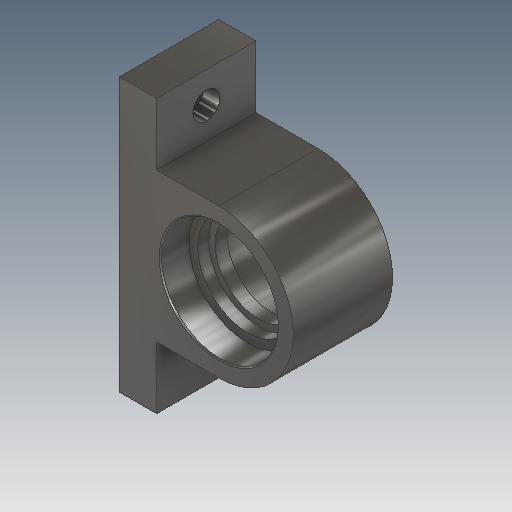
# Autodesk Inventor part: shoulder_joint_fit_v2
Saved by Autodesk Inventor 2021.4 (Build 254397000, 397)
## iProperties
Created: 2020-05-06
Part Number: shoulder_joint_fit_v2
Material: Stahl, hochfest, niedrig legiert
Document SubType Name: Modeling
Designer: Alex
Density: 7.85 g/cm^3
Appearance: Stahl - poliert
Mass: 965.569 g
Surface Area: 266.743 cm^2
Volume: 123.002 cm^3
Author: Alex
Autodesk Inventor part; units mm, degrees
ref_plane "YZ Plane" through (0, 0, 0) normal (1, 0, 0) x (0, 1, 0)
ref_plane "XZ Plane" through (0, 0, 0) normal (0, 1, 0) x (-1, 0, 0)
sketch "Skizze1" plane through (0, 0, 0) normal (0, 0, 1) x (1, 0, 0)
  line L0 (0, 0) -> (55, 0)
  line L1 (55, 0) -> (55, 60)
  line L2 (55, 60) -> (0, 60)
  line L3 (0, 60) -> (0, 0)
  dimension "d0" = 60
  dimension "d1" = 55
  constraints: 8 end point, 2 parallel, 1 horizontal, 1 perpendicular
  measures "d0" distance between parallel lines of L0 L2
  measures "d1" distance of L1.end L2.end
extrude "Grundkörper" add sketch "Skizze1" along normal blind 40
fillet "Konturverrundung" radius 30 2 edges at (55, 60, 20) (55, 0, 20)
sketch "Skizze2" plane through (0, 0, 40) normal (0, 0, 1) x (1, 0, 0)
  point P0 (0, 0)
  point P1 (25, 30)
  point P2 (25, 30)
  constraints: 1 coincident
hole "Durchgangsbohrung 60H7" at (25, 30, 40) direction (0, 0, -1) diameter 55 end through all
sketch "Skizze3" plane through (0, 0, 0) normal (-1, 0, 0) x (0, 0, 1)
  line L0 (0, 0) -> (40, 0) construction
  line L1 (40, 60) -> (40, 0) construction
  line L2 (0, 0) -> (40, 60) construction
  line L3 (0, 60) -> (40, 60) construction
  line L4 (0, 60) -> (40, 0) construction
  line L5 (0, 85) -> (40, 85)
  line L6 (40, 85) -> (40, -25)
  line L7 (40, -25) -> (0, -25)
  line L8 (0, -25) -> (0, 85)
  line L9 (0, 85) -> (40, -25) construction
  line L10 (40, 85) -> (0, -25) construction
  point P0 (20, 30)
  dimension "d16" = 110
  constraints: 16 end point, 3 midpoint, 2 parallel, 1 collinear, 1 horizontal, 1 perpendicular
  measures "d16" distance of L5.end L6.end
extrude "Aufnahmeplatte" add sketch "Skizze3" along normal blind 15
sketch "Skizze4" plane through (0, 0, 0) normal (1, 0, 0) x (0, 0, -1)
  line L0 (-40, 85) -> (0, 85) projected
  line L1 (-20, 85) -> (-20, -25)
  line L2 (-40, -25) -> (0, -25) projected
  line L3 (0, 60) -> (-40, 60) projected
  line L4 (8, 30) -> (-48, 30) projected
  point P0 (0, 0)
  point P1 (-20, 72.5)
  point P2 (-20, -12.5)
  dimension "d26" = 25
  dimension "d27" = 12.5
  constraints: 2 end point, 2 midpoint, 1 point on line, 1 symmetric about line
  measures "d26" distance between parallel lines of L0 L3
  measures "d27" distance from line of point (-20, 72.5) L0
hole "Senkung_Zylinderkopfschraube M6" at (0, 72.5, 20) at (0, -12.5, 20) direction (-1, 0, 0) diameter 6.6 end through all counterbore diameter 11 counterbore depth 6.6 clearance for "Inbusschraube DIN EN ISO 4762" size "M6" standard "DIN"
ref_plane "Konstruktionshilfsebene" through (25, 30, 0) normal (-1, 0, 0) x (0, -1, 0)
ref_plane "Arbeitsebene3" through (55, 30, 0) normal (-1, 0, 0) x (0, -1, 0)
sketch "Skizze6" plane through (25, 30, 0) normal (-1, 0, 0) x (0, -1, 0)
  line L0 (-27.5, 0) -> (-27.5, 40) construction
  line L1 (-6.1835, 0) -> (-3.8165, 0) construction
  line L2 (0, 0) -> (0, 40) construction
  line L3 (-27.5, 40) -> (27.5, 40) construction
  line L4 (-27.5, 40) -> (-23.5, 40)
  line L5 (-23.5, 40) -> (-23.5, 28.5)
  line L6 (-23.5, 28.5) -> (-20, 28.5)
  line L7 (-20, 28.5) -> (-20, 24)
  line L8 (-17.5, 24) -> (-17.5, 19)
  line L9 (-17.5, 19) -> (-21, 19)
  line L10 (-21, 19) -> (-21, 7)
  line L11 (-21, 7) -> (-21, 7)
  line L12 (-22, 6) -> (-22, 0)
  line L13 (27.5, 0) -> (-27.5, 0) construction
  line L14 (-22, 0) -> (-27.5, 0)
  line L15 (-21, 7) -> (-22, 6)
  line L16 (-27.5, 40) -> (-27.5, 0)
  line L17 (-20, 24) -> (-17.5, 24)
  point P0 (30, 0)
  point P1 (-22, 7)
  dimension "d46" = 47
  dimension "d47" = 11.5
  dimension "d48" = 40
  dimension "d49" = 35
  dimension "d52" = 33
  dimension "d53" = 21
  dimension "d54" = 42
  dimension "d55" = 44
  dimension "d57" = 1
  dimension "d58" = 1
  dimension "d79" = 9.5
  dimension "d80" = 16
  constraints: 28 end point, 5 perpendicular, 4 point on line, 3 vertical, 2 horizontal, 2 midpoint, 1 collinear, 1 parallel
  measures "d46" diameter of L5 L2
  measures "d47" distance between parallel lines of L3 L6
  measures "d48" diameter of L7 L2
  measures "d49" diameter of L8 L2
  measures "d52" distance between parallel lines of L11 L3
  measures "d53" distance between parallel lines of L9 L3
  measures "d54" diameter of L10 L2
  measures "d55" diameter of L12 L2
  measures "d57" distance of L11.end point (-22, 7)
  measures "d58" distance of L12.start point (-22, 7)
  measures "d79" distance between parallel lines of L9 L6
  measures "d80" distance between parallel lines of L3 L17
revolve "Lagersitz" add sketch "Skizze6" angle 360 about axis through (25, 30, 0) along (0, 0, 1)
sketch "Skizze8" plane through (0, 0, 0) normal (0, 0, -1) x (-1, 0, 0)
  circle A0 centre (-25, 30) radius 17.5 construction
  line L0 (-25, 60) -> (0, 60) construction
  line L1 (-25, 30) -> (-25, 60) construction
  line L2 (-25, 30) -> (-55, 30) construction
  arc A1 (-25, 60) -> (-25, 0) centre (-25, 30) ccw construction
  circle A2 centre (-25, 30) radius 26 construction
  point P0 (0, 0)
  point P1 (-25, 56)
  point P2 (-51, 30)
  point P3 (-25, 4)
  point P4 (1, 30)
  dimension "d68" = 52
  dimension "d67" = 30
  dimension "d71" = 360
  constraints: 4 end point, 1 coincident, 1 horizontal, 1 point on circle, 1 point on line, 1 vertical, 1 vertical alignment, 7 other
  measures "d67" radius of A1
hole "Gewinde_Keine_ISO Metrisches Profil_2_Winkel(5)" at (25, 56, 0) at (51, 30, 0) at (25, 4, 0) at (-1, 30, 0) direction (0, 0, 1) diameter 1.567 depth 10 tip angle 118 thread size "M2x0.4" class "6H" standard "ISO Metric profile"
chamfer "Gewindesenkung 0.4mm" distance 0.4 angle 45 4 edges at (25, 55.2165, 0) (51, 29.2165, 0) (-1, 29.2165, 0) (25, 3.2165, 0)
chamfer "Fase4" distance 0.5 angle 45 1 edges at (25, 6.5, 40)
equation "\"d27\" = 0.5 * d26"
equation "\"d58\" = d57"
